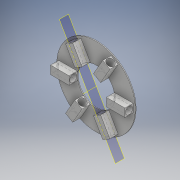
# Autodesk Inventor part: rotor-type2
Saved by Autodesk Inventor 2018 (Build 220112000, 112)
## iProperties
Created: 2025-02-23
Part Number: rotor-type2
Material: Generic
Document SubType Name: Modeling
Designer: neo
Density: 1 g/cm^3
Appearance: Default
Author: neo
Autodesk Inventor part; units mm, degrees
ref_plane "YZ Plane" through (0, 0, 0) normal (1, 0, 0) x (0, 1, 0)
ref_plane "XZ Plane" through (0, 0, 0) normal (0, 1, 0) x (-1, 0, 0)
ref_plane "XY Plane" through (0, 0, 0) normal (0, 0, 1) x (1, 0, 0)
sketch "Sketch1" plane through (0, 0, 0) normal (0, 1, 0) x (-1, 0, 0)
  line L0 (-2.439, 100.9756) -> (-2.439, -121.4634)
  line L1 (89.878, -3.9024) -> (-81.0976, -3.9024)
  line L2 (87.561, 6.0976) -> (42.561, 6.0976)
  line L3 (42.561, 6.0976) -> (42.561, -13.9024)
  line L4 (42.561, -13.9024) -> (87.561, -13.9024)
  line L5 (87.561, -13.9024) -> (87.561, 6.0976)
  line L6 (33.9007, 79.0398) -> (11.4007, 40.0687)
  line L7 (11.4007, 40.0687) -> (28.7212, 30.0687)
  line L8 (28.7212, 30.0687) -> (51.2212, 69.0398)
  line L9 (51.2212, 69.0398) -> (33.9007, 79.0398)
  line L10 (-56.0993, 69.0398) -> (-33.5993, 30.0687)
  line L11 (-33.5993, 30.0687) -> (-16.2788, 40.0687)
  line L12 (-16.2788, 40.0687) -> (-38.7788, 79.0398)
  line L13 (-38.7788, 79.0398) -> (-56.0993, 69.0398)
  line L14 (-92.439, -13.9024) -> (-47.439, -13.9024)
  line L15 (-47.439, -13.9024) -> (-47.439, 6.0976)
  line L16 (-47.439, 6.0976) -> (-92.439, 6.0976)
  line L17 (-92.439, 6.0976) -> (-92.439, -13.9024)
  line L18 (-38.7788, -86.8447) -> (-16.2788, -47.8736)
  line L19 (-16.2788, -47.8736) -> (-33.5993, -37.8736)
  line L20 (-33.5993, -37.8736) -> (-56.0993, -76.8447)
  line L21 (-56.0993, -76.8447) -> (-38.7788, -86.8447)
  line L22 (51.2212, -76.8447) -> (28.7212, -37.8736)
  line L23 (28.7212, -37.8736) -> (11.4007, -47.8736)
  line L24 (11.4007, -47.8736) -> (33.9007, -86.8447)
  line L25 (33.9007, -86.8447) -> (51.2212, -76.8447)
  point P0 (0, 0)
  point P1 (-2.439, -3.9024)
  point P2 (43.7195, 76.0465)
  point P3 (-48.5976, 76.0465)
  point P4 (-94.7561, -3.9024)
  point P5 (-48.5976, -83.8514)
  point P6 (43.7195, -83.8514)
  dimension "d0" = 180
  dimension "d1" = 20
  dimension "d3" = 90
  dimension "d6" = 360
  constraints: 52 end point, 2 horizontal, 2 parallel, 2 point on line, 1 perpendicular, 1 vertical, 56 other
  measures "d0" diameter of L5 L0
  measures "d1" distance between parallel lines of L2 L4
  measures "d3" diameter of L3 L0
extrude "Extrusion1" add sketch "Sketch1" along normal blind 20
sketch "Sketch2" plane through (-11.4007, 0, -47.8736) normal (0.5, 0, 0.8660254) x (0.8660254, 0, -0.5)
  line L0 (-20, 0) -> (0, 0) projected
  line L1 (0, 0) -> (0, 20) projected
  line L2 (-20, 20) -> (0, 20) projected
  line L3 (-20, 0) -> (-20, 20) projected
  line L4 (-20, 20) -> (0, 0)
  line L5 (-20, 20) -> (0, 20) projected
  line L6 (-20, 0) -> (0, 20)
  circle A0 centre (-10, 10) radius 8.75
  point P0 (-14.0635, 0)
  dimension "d10" = 17.5
  constraints: 4 end point, 1 centre point, 1 midpoint, 1 perpendicular
  measures "d10" diameter of A0
extrude "Extrusion2" cut sketch "Sketch2" against normal through all contours A0 L4 L6 | L6 L4 A0 | L4 L6 A0 | A0 L6 L4
pattern_circular "Circular Pattern1" count 6 over 360 about axis through (2.439, 0, -3.9024) along (0, -1, 0) of "Extrusion2"
ref_plane "Work Plane1" through (24.939, 0, -42.8736) normal (-0.8660254, 0, -0.5) x (-0.5, 0, 0.8660254)
sketch "Sketch3" plane through (24.939, 0, -42.8736) normal (-0.8660254, 0, -0.5) x (-0.5, 0, 0.8660254)
  line L0 (45, 26.4) -> (45, -4.4) projected
  line L1 (0, 20) -> (-50, 20)
  line L2 (-50, 20) -> (-50, 22)
  line L3 (-50, 22) -> (0, 22)
  line L4 (0, 22) -> (0, 20)
  line L5 (-8.6603, 20) -> (8.6603, 20) projected
  point P0 (49.5991, 0)
  dimension "d16" = 90
  dimension "d18" = 2
  dimension "d19" = 0
  dimension "d21" = 190
  constraints: 8 end point, 2 parallel, 1 horizontal, 1 perpendicular
  measures "d16" diameter of L4 L0
  measures "d18" distance of L3.end L1.start
  measures "d19" distance between parallel lines of L5 L1
  measures "d21" diameter of L2 L0
revolve "Revolution1" add sketch "Sketch3" angle 360 about axis through (2.439, 0, -3.9024) along (0, -1, 0)
body "Solid1"
